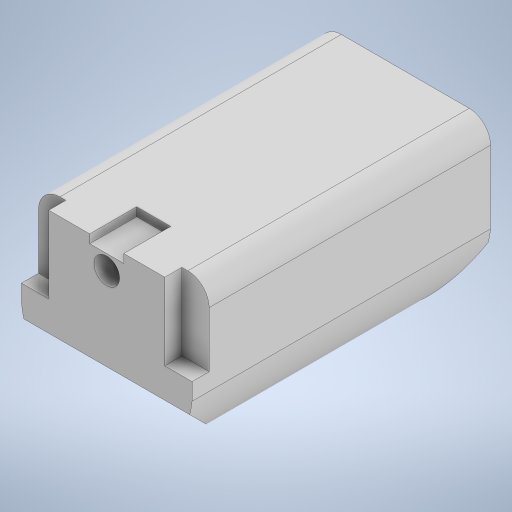
# Autodesk Inventor part: BaseKnuckle
Saved by Autodesk Inventor 2023 (Build 270158000, 158)
## iProperties
Created: 2023-04-06
Part Number: BaseKnuckle
Material: Generic
Document SubType Name: Modeling
Designer: 1senadi
Density: 1 g/cm^3
Appearance: Default
Author: 1senadi
Autodesk Inventor part; units mm, degrees
sketch "Sketch1" plane through (0, 0, 0) normal (0, 1, 0) x (-1, 0, 0)
  line L0 (0, 0) -> (20, 0)
  line L1 (20, 0) -> (20, -20)
  line L2 (20, -20) -> (0, -20)
  line L3 (0, -20) -> (0, 0)
  dimension "d0" = 20
  dimension "d1" = 20
  constraints: 8 end point, 2 parallel, 1 horizontal, 1 perpendicular
  measures "d0" distance of L1.end L2.end
  measures "d1" distance of L0.end L1.end
extrude "Extrusion1" add sketch "Sketch1" along normal blind 35
sketch "Sketch3" plane through (0, 0, 0) normal (1, 0, 0) x (0, 0, -1)
  line L0 (0, 35) -> (20, 35) projected
  line L1 (20, 35) -> (0, 35) projected
  line L2 (20, 35) -> (12.5, 35)
  line L3 (12.5, 35) -> (14, 35)
  line L4 (12.5, 35) -> (11, 35)
  line L5 (14, 35) -> (18.5, 35)
  line L6 (18.5, 35) -> (18.5, 33)
  line L7 (18.5, 33) -> (14, 35)
  line L8 (11, 35) -> (6.5, 35)
  line L9 (6.5, 35) -> (6.5, 33)
  line L10 (6.5, 33) -> (11, 35)
  line L11 (6.5, 33) -> (18.5, 33)
  line L12 (11, 35) -> (11, 33)
  line L13 (14, 35) -> (14, 33)
  point P0 (0, 0)
  dimension "d55" = 7.5
  dimension "d56" = 1.5
  dimension "d57" = 1.5
  dimension "d58" = 4.5
  dimension "d59" = 2
  dimension "d60" = 4.5
  dimension "d61" = 2
  constraints: 24 end point, 7 point on line, 4 perpendicular
  measures "d55" distance of L0.end L2.end
  measures "d56" distance of L2.end L3.end
  measures "d57" distance of L2.end L4.end
  measures "d58" distance of L3.end L5.end
  measures "d59" distance of L5.end L6.end
  measures "d60" distance of L4.end L8.end
  measures "d61" distance of L8.end L9.end
extrude "Extrusion3" cut sketch "Sketch3" against normal blind 3.2 contours L0 L13 L11 L12
sketch "Sketch9" plane through (0, 33, -14) normal (0, 0, 1) x (1, 0, 0)
  line L0 (0, 0) -> (-3.2, 0) projected
  line L1 (-3.2, 2) -> (0, 2) projected
  line L2 (0, 0) -> (-3.2, 0)
  line L3 (-3.2, 0) -> (-3.2, 2)
  line L4 (-3.2, 2) -> (0, 2)
  line L5 (0, 2) -> (0, 0)
  point P0 (0, -33)
  constraints: 8 end point, 2 parallel, 1 horizontal, 1 perpendicular
extrude "Extrusion9" cut sketch "Sketch9" against normal up to surface (6 mm away)
ref_plane "Work Plane1" through (-10, 35, -20) normal (-1, 0, 0) x (0, -1, 0)
sketch "Sketch4" plane through (0, 0, 0) normal (0, -1, 0) x (1, 0, 0)
  line L0 (-20, 0) -> (0, 0) projected
  line L1 (0, -20) -> (-20, -20) projected
  line L2 (0, -20) -> (-20, -20) projected
  line L3 (0, -20) -> (-3.5, -20)
  line L4 (-3.5, -20) -> (-3.5, -13.5)
  line L5 (-3.5, -13.5) -> (-3.5, -11.5)
  line L6 (-3.5, -11.5) -> (-6.5, -11.5)
  line L7 (-6.5, -11.5) -> (-6.5, -13.5)
  line L8 (-6.5, -13.5) -> (-3.5, -13.5)
  line L9 (-10, -20) -> (-10, 0)
  line L10 (-20, 0) -> (0, 0) projected
  line L11 (-16.5, -13.5) -> (-16.5, -11.5)
  line L12 (-16.5, -11.5) -> (-13.5, -11.5)
  line L13 (-13.5, -11.5) -> (-13.5, -13.5)
  line L14 (-13.5, -13.5) -> (-16.5, -13.5)
  dimension "d62" = 3.5
  dimension "d63" = 6.5
  dimension "d64" = 2
  dimension "d65" = 3
  dimension "d66" = 2
  constraints: 22 end point, 4 symmetric about line, 2 midpoint, 2 perpendicular, 2 vertical, 1 point on line
  measures "d62" distance of L1.start L3.end
  measures "d63" distance of L3.end L4.end
  measures "d64" distance of L4.end L5.end
  measures "d65" distance of L5.end L6.end
  measures "d66" distance of L6.end L7.end
extrude "Extrusion4" cut sketch "Sketch4" against normal blind 2.5
fillet "Fillet3" radius 2.5 4 edges at (0, 17.5, 0) (-20, 17.5, 0) (-20, 17.5, -20) (0, 16.5, -20)
sketch "Sketch6" plane through (0, 35, 0) normal (0, 1, 0) x (1, 0, 0)
  line L0 (-2, 0) -> (-18, 0) projected
  line L1 (-10, 0) -> (-10, 20)
  line L2 (-18, 20) -> (-2, 20) projected
  line L3 (-10, 0) -> (-10, 1.25)
  circle A0 centre (-10, 10) radius 8.75
  line L4 (-10, 1.25) -> (-11, 1.25)
  line L5 (-10, 1.25) -> (-9, 1.25)
  line L6 (-10, 1.25) -> (-9, 1.25) construction
  line L7 (-9, 1.25) -> (-9, 20)
  line L8 (-2, 20) -> (-18, 20) projected
  line L9 (-9, 20) -> (-11, 20)
  line L10 (-11, 20) -> (-11, 1.25)
  circle A1 centre (-10, 17.25) radius 1.5
  circle A2 centre (-10, 2.25) radius 1
  point P0 (0, 0)
  point P1 (-11, 18.6927)
  point P2 (-11, 1.3073)
  point P3 (-9, 1.3073)
  point P4 (-9, 18.6927)
  dimension "d40" = 1.25
  dimension "d41" = 1
  dimension "d42" = 1
  dimension "d43" = 0
  dimension "d44" = 90
  dimension "d45" = 2
  dimension "d69" = 3
  dimension "d70" = 2
  dimension "d71" = 0
  dimension "d72" = 0
  dimension "d73" = 0
  constraints: 16 end point, 3 horizontal, 3 midpoint, 3 point on line, 2 centre point, 1 collinear, 1 perpendicular, 4 other
  measures "d40" distance of L1.start L3.end
  measures "d41" distance of L3.end L4.end
  measures "d42" distance of L3.end L5.end
  measures "d43" distance between parallel lines of L5 L6
  measures "d44" angle of L7 L5
  measures "d45" distance of L7.end L9.end
  measures "d69" diameter of A1
  measures "d70" diameter of A2
  measures "d71" distance from line of L1 A2.centre
  measures "d72" distance from line of L1 A1.centre
ref_plane "Work Plane2" through (0, 2, -2) normal (1, 0, 0) x (0, 0, -1)
sketch "Sketch7" plane through (0, 2, -2) normal (1, 0, 0) x (0, 0, -1)
  line L0 (-2, -2) -> (-2, 5.5)
  line L1 (-2, -2) -> (-2, 33) projected
  line L2 (-2, 5.5) -> (5.5, -2)
  line L3 (5.5, -2) -> (-2, -2)
  line L4 (7, -2) -> (7, 0.2) projected
  point P0 (-2, 0)
  point P1 (-2, 31)
  dimension "d36" = 7.5
  dimension "d37" = 45
  constraints: 6 end point, 1 perpendicular, 1 point on line
  measures "d36" distance of L0.start L0.end
  measures "d37" angle of L0 L2
extrude "Extrusion6" cut sketch "Sketch7" against normal up to surface (20 mm away)
extrude "Extrusion7" cut sketch "Sketch6" against normal up to surface (35 mm away) contours A2 L1 | L1 A2 | A1 L10 L1 | L1 A1 L7 | L7 A1 | A1 L10
sketch "Sketch8" plane through (0, 35, 0) normal (0, 1, 0) x (1, 0, 0)
  line L0 (-9, 18.6927) -> (-9, 1.3073) projected
  line L1 (-11, 1.3073) -> (-11, 18.6927) projected
  arc A0 (-11, 1.3073) -> (-9, 1.3073) centre (-10, 10) ccw projected
  arc A1 (-9, 18.6927) -> (-11, 18.6927) centre (-10, 10) ccw projected
  circle A2 centre (-10, 10) radius 8.75
  line L2 (-3.2, 11) -> (0, 11) projected
  line L3 (-20, 11) -> (-16.8, 11) projected
  line L4 (-16.8, 9) -> (-20, 9) projected
  line L5 (0, 9) -> (-3.2, 9) projected
  arc A3 (-20, 9) -> (0, 9) centre (-10, 10.0556) ccw
  line L6 (-3.2, 20) -> (-17.5, 20) projected
  arc A4 (-17.5, 20) -> (-20, 17.5) centre (-17.5, 17.5) ccw projected
  line L7 (-20, 17.5) -> (-20, 2.5) projected
  arc A5 (-20, 2.5) -> (-17.5, 0) centre (-17.5, 2.5) ccw projected
  line L8 (-17.5, 0) -> (-2.5, 0) projected
  arc A6 (-2.5, 0) -> (0, 2.5) centre (-2.5, 2.5) ccw projected
  line L9 (0, 2.5) -> (0, 11) projected
  line L10 (0, 11) -> (-3.2, 11) projected
  line L11 (-3.2, 11) -> (-3.2, 20) projected
  point P0 (0, 0)
  point P1 (-10, 0)
  dimension "d51" = 17.5
  constraints: 2 centre point, 2 point on circle, 1 coincident
  measures "d51" diameter of A2
extrude "Extrusion8" cut sketch "Sketch8" against normal up to surface (35 mm away) contours L9 A6 L8 A3 | A3 L8 A5 L7
mirror "Mirror2" about plane through (-10, 35, -20) normal (-1, 0, 0) of "Extrusion3", "Extrusion9"
ref_plane "Work Plane3" through (-20, 17.5, -9) normal (0, 1, 0) x (-1, 0, 0)
mirror "Mirror3" about plane through (-20, 17.5, -9) normal (0, 1, 0) of "Extrusion6"
sketch "Sketch11" plane through (-3.2, 33, -20) normal (0, 0, -1) x (-1, 0, 0)
  line L0 (0, 2) -> (13.6, 2) projected
  line L1 (5.3, 2) -> (8.3, 2) projected
  line L2 (6.8, 2) -> (12.3, 2) construction
  line L3 (8.8, 2) -> (4.8, 2)
  line L4 (4.8, 2) -> (4.8, -3.5)
  line L5 (4.8, -3.5) -> (8.8, -3.5)
  line L6 (8.8, -3.5) -> (8.8, 2)
  point P0 (-3.2, -33)
  point P1 (6.8, 2)
  point P2 (6.8, 2)
  point P3 (4.8, 2)
  dimension "d76" = 4
  dimension "d77" = 5.5
  dimension "d78" = 0
  dimension "d79" = 0
  constraints: 10 end point, 3 midpoint, 2 horizontal, 2 parallel, 1 perpendicular
  measures "d76" distance of L5.end L4.end
  measures "d77" distance of L4.end L3.end
  measures "d78" distance between parallel lines of L0 L3
  measures "d79" distance of point (6.8, 2) point (6.8, 2)
extrude "Extrusion10" cut sketch "Sketch11" against normal blind 1
body "Solid1"
